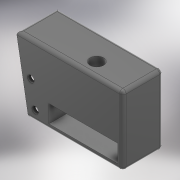
# Autodesk Inventor part: Gripper_Holder_Part3
Saved by Autodesk Inventor 2022 (Build 260153000, 153)
## iProperties
Created: 2023-08-08
Part Number: Gripper_Holder_Part3
Material: Generisch
Document SubType Name: Modeling
Designer: Alsaady
Density: 1 g/cm^3
Appearance: Glatt - Schwarz
Author: Alsaady
## iProperties of the stored document _3D-Druck.ipt
Created: 2023-08-08
Part Number: _3D-Druck
Material: Generisch
Document SubType Name: Modeling
Designer: Alsaady
Density: 1 g/cm^3
Appearance: Vorgabe
Author: Alsaady
Autodesk Inventor part; units mm, degrees
ref_plane "YZ Plane" through (0, 0, 0) normal (1, 0, 0) x (0, 1, 0)
ref_plane "XZ Plane" through (0, 0, 0) normal (0, 1, 0) x (-1, 0, 0)
ref_plane "XY Plane" through (0, 0, 0) normal (0, 0, 1) x (1, 0, 0)
sketch "Skizze1" plane through (0, 0, 0) normal (0, 0, 1) x (1, 0, 0)
  line L0 (20.5, -5.25) -> (-20.5, -5.25)
  line L1 (-20.5, -5.25) -> (-20.5, 5.25)
  line L2 (-20.5, 5.25) -> (20.5, 5.25)
  line L3 (20.5, 5.25) -> (20.5, -5.25)
  line L4 (20.5, -5.25) -> (-20.5, 5.25) construction
  line L5 (-20.5, -5.25) -> (20.5, 5.25) construction
  line L6 (-22.5, -8.25) -> (-39.9555, -8.25)
  line L7 (-39.9555, -8.25) -> (-39.9555, 33.1575)
  line L8 (-39.9555, 33.1575) -> (-22.5, 33.1575)
  line L9 (-22.5, 33.1575) -> (-22.5, -8.25)
  line L10 (-22.5, 33.1575) -> (23.5, 33.1575)
  line L11 (23.5, 33.1575) -> (23.5, -8.25)
  line L12 (23.5, -8.25) -> (-22.5, -8.25)
  line L13 (-22.5, -8.25) -> (-22.5, 33.1575)
  line L14 (-22.5, -8.25) -> (-39.9555, -8.25)
  line L15 (-22.5, 30.1575) -> (-39.9555, 30.1575)
  line L16 (-22.5, -8.25) -> (-29.2723, 30.1575)
  line L17 (-32.6543, -8.25) -> (-39.9555, 33.1575)
  line L18 (-36.3049, 12.4538) -> (-25.8861, 10.9538) construction
  line L19 (-34.3494, 30.1575) -> (-27.5771, -8.25) construction
  circle A0 centre (-31.2443, 12.5475) radius 2
  circle A1 centre (-28.6396, -2.2246) radius 2
  line L20 (-29.2723, 30.1575) -> (-39.9555, 28.2738)
  line L21 (-22.5, -8.25) -> (-22.5, -8.25)
  point P0 (0, 0)
  point P1 (-32.6543, -8.25)
  point P2 (-39.4265, 30.1575)
  point P3 (-31.0955, 11.7038)
  point P4 (-39.1204, 28.421)
  point P5 (-32.334, -7.473)
  dimension "d0" = 10.5
  dimension "d1" = 41
  dimension "d2" = 3
  dimension "d3" = 3
  dimension "d4" = 3
  dimension "d6" = 10
  dimension "d7" = 10
  dimension "d16" = 4
  dimension "d18" = 15
  dimension "d21" = 39
  dimension "d23" = 17
  dimension "d24" = 7
  dimension "d29" = 2
  constraints: 44 end point, 14 point on line, 10 parallel, 5 midpoint, 5 perpendicular, 3 horizontal, 2 centre point, 1 equal radius
  measures "d0" distance of L2.end L0.start
  measures "d1" distance of L0.start L0.end
  measures "d2" distance between parallel lines of L12 L0
  measures "d3" horizontal distance of L11.end L0.start
  measures "d4" distance between parallel lines of L15 L8
  measures "d6" angle of L13 L16
  measures "d7" distance between parallel lines of L16 L17
  measures "d16" diameter of A0
  measures "d18" distance of A0.centre A1.centre
  measures "d21" distance of L6.start L16.end
  measures "d23" distance from line of L20 A0.centre
  measures "d24" distance from line of L21 A1.centre
  measures "d29" horizontal distance of L6.start L0.end
extrude "Extrusion1" add sketch "Skizze1" along normal blind 20 contours L16 L15 L9 | L9 L10 L11 L12 | L15 L17 L8 L9 | L20 L17 L15
extrude "Extrusion2" add sketch "Skizze1" against normal blind 2 contours L0 L1 L2 L3 | L16 L15 L9 | L9 L10 L11 L12 | L6 L17 L20 L16 | L15 L17 L8 L9 | L20 L17 L15
sketch "Skizze2" plane through (0, 0, 20) normal (0, 0, 1) x (1, 0, 0)
  line L0 (-39.9555, 33.1575) -> (-39.1204, 28.421) projected
  line L1 (23.5, -8.25) -> (23.5, 33.1575) projected
  line L2 (23.5, 33.1575) -> (-39.9555, 33.1575) projected
  line L3 (20.5, -5.25) -> (-20.5, -5.25) projected
  line L4 (-20.5, -5.25) -> (-20.5, 5.25) projected
  line L5 (-20.5, 5.25) -> (20.5, 5.25) projected
  line L6 (20.5, 5.25) -> (20.5, -5.25) projected
  line L7 (-39.9555, 33.1575) -> (-32.8306, -7.25) projected
  line L8 (-39.9555, 33.1575) -> (-32.8306, -7.25)
  circle A0 centre (-28.6396, -2.2246) radius 2 projected
  circle A1 centre (-31.2443, 12.5475) radius 2 projected
  line L9 (-39.1204, 28.421) -> (-29.2723, 30.1575) projected
  line L10 (-29.2723, 30.1575) -> (-22.5, -8.25) projected
  line L11 (-22.5, -8.25) -> (23.5, -8.25) projected
  line L12 (-39.1204, 28.421) -> (-29.2723, 30.1575) projected
  line L13 (-39.1204, 28.421) -> (-32.6543, -8.25) projected
  line L14 (-32.6543, -8.25) -> (-22.5, -8.25) projected
  line L15 (-29.2723, 30.1575) -> (-22.5, -8.25) projected
  circle A2 centre (-28.6396, -2.2246) radius 2 projected
  circle A3 centre (-31.2443, 12.5475) radius 2 projected
  point P0 (0, 0)
  point P1 (-39.1307, 33.9543)
  point P2 (-39.1307, 33.9543)
  point P3 (-32.6543, -7.25)
  point P4 (-32.8306, -7.25)
  constraints: 2 end point, 2 other
extrude "Extrusion3" add sketch "Skizze2" along normal blind 2
fillet "Rundung1" radius 2 9 edges at (-8.2278, 33.1575, 22) (23.5, 12.4538, 22) (23.5, 12.4538, -2) (23.5, 33.1575, 10) (23.5, -8.25, 10) (-4.5771, -8.25, -2) (-8.2278, 33.1575, -2) (-4.5771, -8.25, 22) (-39.9555, 33.1575, 10)
sketch "Skizze3" plane through (-32.6543, -7.5, 20) normal (0, -1, 0) x (1, 0, 0)
  line L0 (53.1543, -20) -> (53.1543, 2) projected
  line L1 (53.1543, -9) -> (0, -9)
  line L2 (0, -20) -> (0, 0) projected
  line L3 (53.1543, 2) -> (12.1543, 2) projected
  line L4 (32.6543, -20) -> (32.6543, 2)
  circle A0 centre (32.6543, -9) radius 2
  dimension "d25" = 4
  constraints: 4 end point, 3 midpoint, 1 centre point, 1 horizontal, 1 point on line
  measures "d25" diameter of A0
extrude "Extrusion4" [suppressed]
fillet "Rundung2" [suppressed]
sketch "Skizze5" plane through (-22.5, -8.25, 20) normal (0, -1, 0) x (1, 0, 0)
  line L0 (43, -20) -> (2, -20) projected
  line L1 (2, -20) -> (2, 2) projected
  line L2 (43, -20) -> (43, 2) projected
  line L3 (22.5, -14) -> (22.5, 2) construction
  line L4 (-17.072, 2) -> (44, 2) projected
  circle A0 centre (22.5, -6) radius 2
  line L5 (43, 2) -> (2, 2) projected
  line L6 (2, -6) -> (43, -6) construction
  dimension "d34" = 4
  dimension "d45" = 16
  constraints: 4 end point, 3 point on line, 2 midpoint, 1 centre point, 1 coincident, 1 horizontal, 1 parallel
  measures "d34" diameter of A0
  measures "d45" distance of L3.start L3.end
extrude "Extrusion6" cut sketch "Skizze5" against normal through all contours A0
fillet "Rundung3" [suppressed]
fillet "Rundung4" radius 3 2 edges at (-33.2443, 12.5475, -2) (-30.6396, -2.2246, -2)
extrude "Extrusion7" add sketch "Skizze5" against normal up to surface (3 mm away) contours A0
sketch "Skizze6" plane through (-37.572, 33.1575, 0) normal (0, 1, 0) x (1, 0, 0)
  circle A0 centre (37.572, -14) radius 2 projected
  circle A1 centre (37.572, -14) radius 2 projected
  circle A2 centre (37.572, -14) radius 4
  point P0 (37.572, 0)
  dimension "d40" = 8
  constraints: 1 centre point, 1 coincident
  measures "d40" diameter of A2
extrude "Extrusion8" cut sketch "Skizze6" against normal blind 10
sketch "Skizze7" plane through (0, 0, 0) normal (0, 0, 1) x (1, 0, 0)
  line L0 (20.5, 5.25) -> (20.5, -5.25) projected
  line L1 (-20.5, 5.25) -> (20.5, 5.25) projected
  line L2 (-20.5, -5.25) -> (-20.5, 5.25) projected
  line L3 (20.5, -5.25) -> (-20.5, -5.25) projected
  point P0 (0, 0)
extrude "Extrusion9" add sketch "Skizze7" along normal blind 10
sketch "Skizze8" plane through (-20.5, 5.25, 22) normal (0, -1, 0) x (1, 0, 0)
  circle A0 centre (20.5, -8) radius 2 projected
  line L0 (24.8301, -8) -> (22.6651, -11.75)
  line L1 (22.6651, -11.75) -> (18.3349, -11.75)
  line L2 (18.3349, -11.75) -> (16.1699, -8)
  line L3 (16.1699, -8) -> (18.3349, -4.25)
  line L4 (18.3349, -4.25) -> (22.6651, -4.25)
  line L5 (22.6651, -4.25) -> (24.8301, -8)
  line L6 (0, -12) -> (41, -12) projected
  point P0 (20.5, -22)
  dimension "d46" = 7.5
  constraints: 12 end point, 1 coincident, 1 parallel, 13 other
  measures "d46" distance between parallel lines of L4 L1
extrude "Extrusion10" cut sketch "Skizze8" against normal blind 5
equation "\"d3\" = d2"
equation "\"d4\" = d2"
